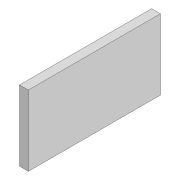
# Autodesk Inventor part: Part1String
Saved by Autodesk Inventor 2020.2 (Build 242310000, 310)
## iProperties
Created: 2020-02-15
Part Number: Part1String
Material: Generic
Document SubType Name: Modeling
Designer: Yash
Density: 1 g/cm^3
Appearance: Default
Author: Yash
Autodesk Inventor part; units mm, degrees
ref_plane "YZ Plane" through (0, 0, 0) normal (1, 0, 0) x (0, 1, 0)
ref_plane "XZ Plane" through (0, 0, 0) normal (0, 1, 0) x (-1, 0, 0)
ref_plane "XY Plane" through (0, 0, 0) normal (0, 0, 1) x (1, 0, 0)
sketch "Sketch1" plane through (0, 0, 0) normal (1, 0, 0) x (0, 1, 0)
  line L0 (4.4552, 9.6275) -> (-75.5448, 9.6275)
  line L1 (-75.5448, 9.6275) -> (-75.5448, -140.3725)
  line L2 (-75.5448, -140.3725) -> (4.4552, -140.3725)
  line L3 (4.4552, -140.3725) -> (4.4552, 9.6275)
  point P0 (0, 0)
  dimension "d0" = 80
  dimension "d1" = 150
  constraints: 8 end point, 2 parallel, 1 horizontal, 1 perpendicular
  measures "d0" distance of L2.end L1.end
  measures "d1" distance of L1.end L0.end
extrude "Extrusion1" add sketch "Sketch1" along normal blind 10
body "Solid1"
